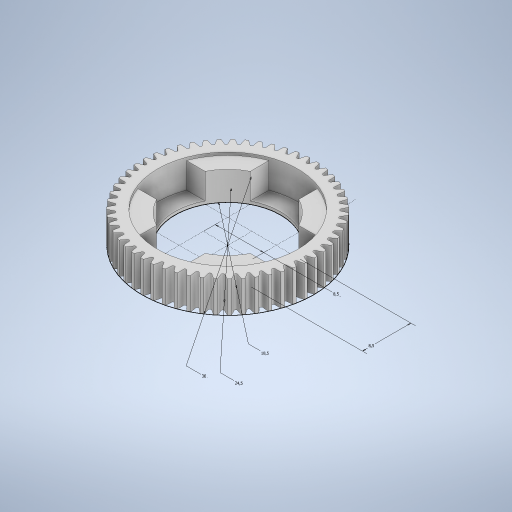
# Autodesk Inventor part: Gear2
Saved by Autodesk Inventor 2024 (Build 280153000, 153)
## iProperties
Created: 2024-10-01
Part Number: Gear2
Material: Типовые
Document SubType Name: Modeling
Designer: fm
Density: 1 g/cm^3
Appearance: По умолчанию
Author: fm
Autodesk Inventor part; units mm, degrees
ref_plane "YZ Plane" through (0, 0, 0) normal (1, 0, 0) x (0, 1, 0)
ref_plane "XZ Plane" through (0, 0, 0) normal (0, 1, 0) x (-1, 0, 0)
ref_plane "XY Plane" through (0, 0, 0) normal (0, 0, 1) x (1, 0, 0)
sketch "Эскиз1" plane through (0, 0, 0) normal (0, 1, 0) x (-1, 0, 0)
  arc A0 (-4.25, 8.2158) -> (4.25, 8.2158) centre (0, 0) ccw
  circle A1 centre (0, 0) radius 12.25
  line L0 (4.25, -17.0887) -> (4.25, -11.4891) construction
  line L1 (-4.25, -18.1421) -> (-4.25, -11.4891) construction
  line L2 (4.25, 0) -> (-4.25, 0) construction
  line L3 (-4.25, 8.2158) -> (-4.25, 11.4891)
  line L4 (-4.25, 11.4891) -> (-4.25, 12.4654) construction
  line L5 (4.25, 8.2158) -> (4.25, 11.4891)
  line L6 (4.25, 11.4891) -> (4.25, 11.412) construction
  line L7 (4.25, -11.4891) -> (4.25, -8.2158)
  line L8 (4.25, -8.2158) -> (4.25, 8.2158) construction
  line L9 (-4.25, -11.4891) -> (-4.25, -8.2158)
  line L10 (-4.25, -8.2158) -> (-4.25, 8.2158) construction
  arc A2 (4.25, 8.2158) -> (-4.25, 8.2158) centre (0, 0) ccw
  circle A3 centre (0, 0) radius 15
  line L11 (-8.2158, -4.25) -> (-11.4891, -4.25)
  line L12 (-8.2158, 4.25) -> (-11.4891, 4.25)
  line L13 (11.4891, 4.25) -> (8.2158, 4.25)
  line L14 (8.2158, 4.25) -> (-8.2158, 4.25) construction
  line L15 (11.4891, -4.25) -> (8.2158, -4.25)
  line L16 (8.2158, -4.25) -> (-8.2158, -4.25) construction
  line L17 (0, -4.25) -> (0, 4.25) construction
  spline S0 degree 3 poles (0.6172, -14.9873) (0.6046, -14.9624) (0.5793, -14.9126) (0.5428, -14.8372) (0.5072, -14.7613) (0.4728, -14.6849) (0.4396, -14.608) (0.4076, -14.5306) (0.3768, -14.4527) (0.3475, -14.3742) (0.3195, -14.2952) (0.2932, -14.2157) (0.2681, -14.1358) (0.2517, -14.0751) (0.2397, -14.035) (0.2324, -14.0153) (0.224, -13.9961) (0.2141, -13.9777) (0.2027, -13.96) (0.1898, -13.9435) (0.1753, -13.9284) (0.1594, -13.9148) (0.1422, -13.9026) (0.1236, -13.8929) (0.1044, -13.8846) (0.0841, -13.8792) (0.0635, -13.8753) (0.0355, -13.8743) (0.0007, -13.8749) (-0.0342, -13.8743) (-0.0622, -13.8753) (-0.0828, -13.8792) (-0.1031, -13.8846) (-0.1223, -13.8929) (-0.1409, -13.9027) (-0.1581, -13.9148) (-0.174, -13.9284) (-0.1885, -13.9435) (-0.2014, -13.9601) (-0.2128, -13.9777) (-0.2227, -13.9962) (-0.2311, -14.0154) (-0.2384, -14.035) (-0.2504, -14.0751) (-0.2668, -14.1358) (-0.2918, -14.2157) (-0.3182, -14.2953) (-0.3461, -14.3743) (-0.3755, -14.4527) (-0.4062, -14.5307) (-0.4382, -14.6081) (-0.4715, -14.685) (-0.5059, -14.7614) (-0.5414, -14.8372) (-0.5779, -14.9126) (-0.6032, -14.9624) (-0.6158, -14.9874) knots 0 0 0 0 0.031252 0.062505 0.093757 0.125009 0.156261 0.187514 0.218766 0.250018 0.28127 0.312522 0.343774 0.375026 0.382839 0.39065 0.398461 0.406273 0.414085 0.421897 0.429707 0.437515 0.445326 0.453135 0.460945 0.468754 0.476564 0.484374 0.5 0.515626 0.523436 0.531246 0.539055 0.546865 0.554674 0.562485 0.570293 0.578103 0.585915 0.593727 0.601539 0.60935 0.617161 0.624974 0.656226 0.687478 0.71873 0.749982 0.781234 0.812486 0.843739 0.874991 0.906243 0.937495 0.968748 1 1 1 1
  point P0 (0.5796, -14.9125)
  point P1 (0.543, -14.8371)
  point P2 (0.5074, -14.7612)
  point P3 (0.473, -14.6848)
  point P4 (0.4398, -14.6079)
  point P5 (0.4078, -14.5305)
  point P6 (0.3771, -14.4526)
  point P7 (0.3477, -14.3741)
  point P8 (0.3198, -14.2952)
  point P9 (0.2934, -14.2157)
  point P10 (0.2686, -14.1356)
  point P11 (0.2457, -14.0551)
  point P12 (0.2395, -14.035)
  point P13 (0.2322, -14.0154)
  point P14 (0.2237, -13.9963)
  point P15 (0.2139, -13.9778)
  point P16 (0.2025, -13.9602)
  point P17 (0.1896, -13.9437)
  point P18 (0.1751, -13.9286)
  point P19 (0.1592, -13.915)
  point P20 (0.142, -13.903)
  point P21 (0.1235, -13.8932)
  point P22 (0.1042, -13.8851)
  point P23 (0.0841, -13.8795)
  point P24 (0.0634, -13.8758)
  point P25 (0.0425, -13.8747)
  point P26 (0.0007, -13.8747)
  point P27 (-0.0412, -13.8747)
  point P28 (-0.0621, -13.8758)
  point P29 (-0.0828, -13.8795)
  point P30 (-0.1029, -13.8851)
  point P31 (-0.1222, -13.8932)
  point P32 (-0.1407, -13.9031)
  point P33 (-0.1579, -13.915)
  point P34 (-0.1737, -13.9287)
  point P35 (-0.1883, -13.9438)
  point P36 (-0.2012, -13.9602)
  point P37 (-0.2125, -13.9778)
  point P38 (-0.2224, -13.9963)
  point P39 (-0.2309, -14.0154)
  point P40 (-0.2382, -14.0351)
  point P41 (-0.2443, -14.0551)
  point P42 (-0.2673, -14.1356)
  point P43 (-0.292, -14.2157)
  point P44 (-0.3184, -14.2952)
  point P45 (-0.3464, -14.3742)
  point P46 (-0.3757, -14.4526)
  point P47 (-0.4064, -14.5306)
  point P48 (-0.4384, -14.608)
  point P49 (-0.4717, -14.6849)
  point P50 (-0.5061, -14.7613)
  point P51 (-0.5416, -14.8371)
  point P52 (-0.5782, -14.9125)
  dimension "d1" = 24.5
  dimension "d0" = 18.5
  dimension "d2" = 8.5
  dimension "d3" = 30
  dimension "d4" = 8.5
  constraints: 36 end point, 12 point on circle, 11 vertical, 6 horizontal, 6 midpoint, 5 coincident, 5 perpendicular, 4 point on line, 3 centre point, 65 other
  measures "d0" diameter of A0
  measures "d2" distance of L2.start L2.end
  measures "d3" diameter of A3
  measures "d4" distance between parallel lines of L14 L16
extrude "Выдавливание1" add sketch "Эскиз1" along normal blind 0.5 contours A0 L12 A1 L3 | L3 A1 L5 A2 | A0 L11 A1 L12 | L5 A1 L13 A0 | A0 L9 A1 L11 | L13 A1 L15 A0 | A0 L7 A1 L9 | L15 A1 L7 A0 | A3 S0 | S0 A3
extrude "Выдавливание2" add sketch "Эскиз1" along normal blind 4.5 from surface at 0.5 contours A0 L12 A1 L3 | L5 A1 L13 A0 | A0 L9 A1 L11 | L15 A1 L7 A0 | A3 S0 | S0 A3
extrude "Выдавливание3" add sketch "Эскиз1" along normal blind 0.5 from surface at 5
extrude "Выдавливание4" cut sketch "Эскиз1" along normal through all contours S0 A3 picked at (0.0501, -14.4988)
pattern_circular "Круговой массив1" count 55 over 360 about axis through (0, 0, 0) along (0, 1, 0) of "Выдавливание4"
